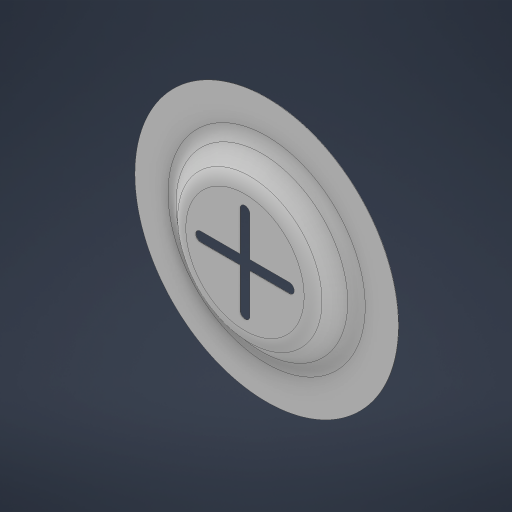
# Autodesk Inventor part: bat_contacts_v2_contact_round
Saved by Autodesk Inventor 2024.3 (Build 283343010, 343A)
## iProperties
Created: 2025-05-14
Part Number: bat_contacts_v2_contact_round
Material: Generisch
Document SubType Name: Sheet Metal
Designer: David
Density: 1 g/cm^3
Sheet Metal Rule: Standard_mm
Appearance: Vorgabe
Author: David
Autodesk Inventor part; units mm, degrees
ref_plane "YZ Plane" through (0, 0, 0) normal (1, 0, 0) x (0, 1, 0)
ref_plane "XZ Plane" through (0, 0, 0) normal (0, 1, 0) x (-1, 0, 0)
ref_plane "XY Plane" through (0, 0, 0) normal (0, 0, 1) x (1, 0, 0)
sketch "Skizze1" plane through (0, 0, 0) normal (0, 0, 1) x (1, 0, 0)
  line L0 (0, 0) -> (0, -0.02)
  line L1 (0, -0.02) -> (-3, -0.02)
  arc A0 (-3.6591, 0.2279) -> (-3, -0.02) centre (-3, 0.98) ccw
  line L2 (-3.6591, 0.2279) -> (-4.3541, 0.837)
  arc A1 (-4.3541, 0.837) -> (-5, 1.08) centre (-5, 0.1) ccw
  line L3 (-5, 1.08) -> (-6.68, 1.08)
  line L4 (-6.68, 1.08) -> (-6.68, 1.1)
  line L5 (-6.68, 1.1) -> (-5, 1.1)
  arc A2 (-4.3409, 0.8521) -> (-5, 1.1) centre (-5, 0.1) ccw
  line L6 (-4.3409, 0.8521) -> (-3.6459, 0.243)
  line L7 (-3, 0) -> (0, 0)
  arc A3 (-3.6459, 0.243) -> (-3, 0) centre (-3, 0.98) ccw
  dimension "d0" = 0.02
  dimension "d2" = 10
  dimension "d3" = 0.02
  dimension "d4" = 1
  dimension "d5" = 1.1
  dimension "d6" = 6
  constraints: 16 end point, 8 point on circle, 7 tangent, 4 centre point, 3 parallel, 3 perpendicular, 1 coincident, 1 concentric, 1 equal radius, 1 vertical
  measures "d0" distance between parallel lines of L1 L7
  measures "d2" diameter of L3.start L0
  measures "d3" distance between parallel lines of L3 L5
  measures "d4" radius of A0
  measures "d5" distance between parallel lines of L1 L3
  measures "d6" diameter of L7.start L0
revolve "Umdrehung1" add sketch "Skizze1" angle 360 about axis through (0, 0, 0) along (0, -1, 0)
sketch "Skizze2" plane through (0, -0.02, 0) normal (0, -1, 0) x (1, 0, 0)
  line L0 (0, 0) -> (0, 2.5)
  line L1 (0, 2.5) -> (0.25, 2.5)
  line L2 (0.25, 2.5) -> (0.25, 0.25)
  line L3 (0.25, 0.25) -> (2.5, 0.25)
  line L4 (2.5, 0.25) -> (2.5, 0)
  line L5 (2.5, 0) -> (0, 0)
  arc A0 (2.5, 0) -> (2.25, 0.25) centre (2.25, 0) ccw
  arc A1 (0.25, 2.25) -> (0, 2.5) centre (0, 2.25) ccw
  arc A2 (-2.25, 0.25) -> (-2.5, 0) centre (-2.25, 0) ccw
  line L6 (-2.5, 0.25) -> (-0.25, 0.25)
  line L7 (-0.25, 2.5) -> (0, 2.5)
  arc A3 (0, 2.5) -> (-0.25, 2.25) centre (0, 2.25) ccw
  line L8 (-0.25, 0.25) -> (-0.25, 2.5)
  line L9 (-2.5, 0) -> (-2.5, 0.25)
  arc A4 (-0.25, -2.25) -> (0, -2.5) centre (0, -2.25) ccw
  line L10 (-0.25, -2.5) -> (-0.25, -0.25)
  line L11 (-2.5, -0.25) -> (-2.5, 0)
  arc A5 (-2.5, 0) -> (-2.25, -0.25) centre (-2.25, 0) ccw
  line L12 (-0.25, -0.25) -> (-2.5, -0.25)
  line L13 (0, -2.5) -> (-0.25, -2.5)
  arc A6 (2.25, -0.25) -> (2.5, 0) centre (2.25, 0) ccw
  line L14 (2.5, -0.25) -> (0.25, -0.25)
  line L15 (0.25, -2.5) -> (0, -2.5)
  arc A7 (0, -2.5) -> (0.25, -2.25) centre (0, -2.25) ccw
  line L16 (0.25, -0.25) -> (0.25, -2.5)
  line L17 (2.5, 0) -> (2.5, -0.25)
  point P0 (0, 2.5)
  point P1 (-2.5, 0)
  point P2 (0, -2.5)
  point P3 (2.5, 0)
  dimension "d8" = 5
  dimension "d9" = 0.5
  dimension "d12" = 360
  constraints: 36 end point, 16 point on circle, 8 centre point, 8 point on line, 7 perpendicular, 4 tangent, 1 vertical, 61 other
  measures "d8" diameter of L4 L0
  measures "d9" diameter of L2 L0
extrude "Extrusion1" cut sketch "Skizze2" against normal through all contours L5 A6 L14 L16 A7 A4 L10 L12 A5 A2 L6 L8 A3 L0 | L0 A1 L2 L3 A0 L5
equation "\"d3\" = d0"
equation "\"Biegeradius\" = Stärke"
equation "\"BreiteBiegungsfreistellung\" = Stärke"
equation "\"TiefeBiegungsfreistellung\" = 0.5 * Stärke"
equation "\"GrößeEckenfreistellung\" = 4 * Stärke"
equation "\"MinimalRest\" = 2 * Stärke"
equation "\"Übergangsradius\" = Biegeradius"
equation "\"JacobiRadiusGröße\" = Biegeradius"
equation "\"Abstandsgröße\" = Stärke"
equation "\"Stärke\" = 0.5"
